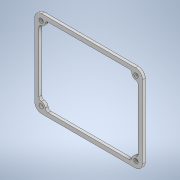
# Autodesk Inventor part: Trippeldekker_Midtre plate
Saved by Autodesk Inventor 2022 (Build 260153000, 153)
## iProperties
Created: 2021-08-24
Part Number: Trippeldekker_Midtre plate
Material: Generic
Document SubType Name: Modeling
Designer: jonar
Density: 1 g/cm^3
Appearance: Default
Author: jonar
Autodesk Inventor part; units mm, degrees
ref_plane "YZ Plane" through (0, 0, 0) normal (1, 0, 0) x (0, 1, 0)
ref_plane "XZ Plane" through (0, 0, 0) normal (0, 1, 0) x (-1, 0, 0)
ref_plane "XY Plane" through (0, 0, 0) normal (0, 0, 1) x (1, 0, 0)
sketch "card+border" plane through (0, 0, 0) normal (0, 0, 1) x (1, 0, 0)
  line L0 (-59.3579, 68.5808) -> (-59.3579, 10.0008)
  line L1 (-59.3579, 10.0008) -> (14.2921, 10.0008)
  line L2 (14.2921, 10.0008) -> (14.2921, 68.5808)
  line L3 (14.2921, 68.5808) -> (-59.3579, 68.5808)
  circle A0 centre (11.6671, 65.9558) radius 1.575
  circle A1 centre (11.6671, 12.6258) radius 1.575
  circle A2 centre (-56.7329, 65.9558) radius 1.575
  circle A3 centre (-56.7329, 12.6258) radius 1.575
  line L4 (-61.3579, 70.5808) -> (-61.3579, 8.0008)
  line L5 (-61.3579, 8.0008) -> (16.2921, 8.0008)
  line L6 (16.2921, 8.0008) -> (16.2921, 70.5808)
  line L7 (16.2921, 70.5808) -> (-61.3579, 70.5808)
  line L8 (-58.3579, 67.5808) -> (13.2921, 67.5808)
  line L9 (13.2921, 67.5808) -> (13.2921, 11.0008)
  line L10 (13.2921, 11.0008) -> (-58.3579, 11.0008)
  line L11 (-58.3579, 11.0008) -> (-58.3579, 67.5808)
  circle A4 centre (-56.7329, 65.9558) radius 3
  circle A5 centre (11.6671, 65.9558) radius 3
  circle A6 centre (11.6671, 12.6258) radius 3
  circle A7 centre (-56.7329, 12.6258) radius 3
  point P0 (0, 0)
  point P1 (-54.2111, 67.5808)
  point P2 (9.1454, 67.5808)
  point P3 (13.2921, 63.434)
  point P4 (13.2921, 15.1475)
  point P5 (9.1454, 11.0008)
  point P6 (-54.2111, 11.0008)
  point P7 (-58.3579, 15.1475)
  point P8 (-58.3579, 63.434)
  dimension "d1" = 58.58
  dimension "d2" = 73.65
  dimension "d4" = 2.625
  dimension "d5" = 3.15
  dimension "d31" = 2.625
  dimension "d32" = 2.625
  dimension "d33" = 2.625
  dimension "d34" = 3.15
  dimension "d35" = 2
  dimension "d36" = 3
  dimension "d37" = 3
  dimension "d38" = 3
  dimension "d39" = 3
  dimension "d40" = 6
  dimension "d41" = 6
  dimension "d42" = 6
  dimension "d43" = 6
  constraints: 24 end point, 8 centre point, 5 perpendicular, 4 coincident, 2 parallel, 1 horizontal, 1 vertical, 3 other
  measures "d1" distance of L1.end L2.end
  measures "d2" distance of L2.end L0.start
  measures "d4" distance from line of L2 A0.centre
  measures "d5" diameter of A0
  measures "d31" distance from line of L3 A0.centre
  measures "d32" distance from line of L3 A2.centre
  measures "d33" distance from line of L0 A2.centre
  measures "d34" diameter of A2
  measures "d35" distance between parallel lines of L3 L7
  measures "d36" distance between parallel lines of L6 L9
  measures "d37" distance between parallel lines of L4 L11
  measures "d38" distance between parallel lines of L5 L10
  measures "d39" distance between parallel lines of L8 L7
  measures "d40" diameter of A4
  measures "d41" diameter of A5
  measures "d42" diameter of A6
  measures "d43" diameter of A7
extrude "Middle wall" add sketch "card+border" along normal blind 2 contours L3 A4 L0 | A4 L3 L8 L11 L0 | L0 A4 | A4 L3 | A4 L11 A7 L0 | L3 A5 L8 A4 | A7 L11 L10 L1 L0 | L0 A7 | L11 L8 A4 | A5 L3 | L3 A5 L2 L9 L8 | A7 L1 L0 | A7 L10 L11 | L3 L2 A5 | L8 L9 A5 | L1 A7 | A5 L2 | A5 L2 A6 L9 | A7 L10 A6 L1 | A6 L2 L1 L10 L9 | L9 L10 A6 | L1 A6 | A6 L2 | A6 L2 L1 | L7 L6 L5 L4
fillet "Skruehull suport" radius 2 8 edges at (9.1454, 67.5808, 1) (13.2921, 63.434, 1) (-58.3579, 63.434, 1) (-54.2111, 67.5808, 1) (-54.2111, 11.0008, 1) (-58.3579, 15.1475, 1) (13.2921, 15.1475, 1) (9.1454, 11.0008, 1)
fillet "Kantutjevning" radius 5 4 edges at (16.2921, 70.5808, 1) (-61.3579, 70.5808, 1) (-61.3579, 8.0008, 1) (16.2921, 8.0008, 1)
body "Solid2"
